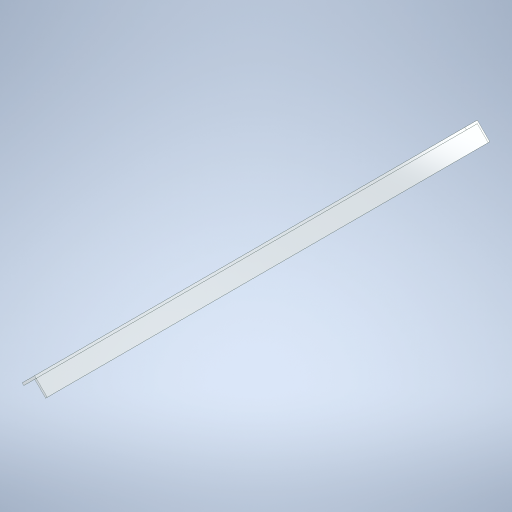
# Autodesk Inventor part: Ridge_Vent
Saved by Autodesk Inventor 2024 (Build 280153000, 153)
## iProperties
Created: 2023-05-20
Part Number: Ridge_Vent
Material: ABS Plastic
Document SubType Name: Modeling
Designer: Tom
Density: 1.06 g/cm^3
Appearance: Clear
Author: Tom
Autodesk Inventor part; units mm, degrees
ref_plane "YZ Plane" through (0, 0, 0) normal (1, 0, 0) x (0, 1, 0)
ref_plane "XZ Plane" through (0, 0, 0) normal (0, 1, 0) x (-1, 0, 0)
ref_plane "XY Plane" through (0, 0, 0) normal (0, 0, 1) x (1, 0, 0)
sketch "Sketch1" plane through (0, 0, 0) normal (0, 0, 1) x (1, 0, 0)
  line L0 (0, 0) -> (-215.5261, -215.5261)
  line L1 (-215.5261, -215.5261) -> (-188.5854, -242.4669)
  line L2 (-188.5854, -242.4669) -> (0, -53.8815)
  line L3 (0, -53.8815) -> (188.5854, -242.4669)
  line L4 (188.5854, -242.4669) -> (215.5261, -215.5261)
  line L5 (215.5261, -215.5261) -> (0, 0)
  line L6 (188.5854, -242.4669) -> (-188.5854, -242.4669)
  dimension "d0" = 38.1
  dimension "d1" = 304.8
  constraints: 14 end point, 7 perpendicular, 1 horizontal
  measures "d0" distance between parallel lines of L0 L2
  measures "d1" distance of L4.end L0.start
extrude "Extrusion1" add sketch "Sketch1" along normal blind 7620 contours L5 L4 L3 L2 L1 L0
body "Solid1"
